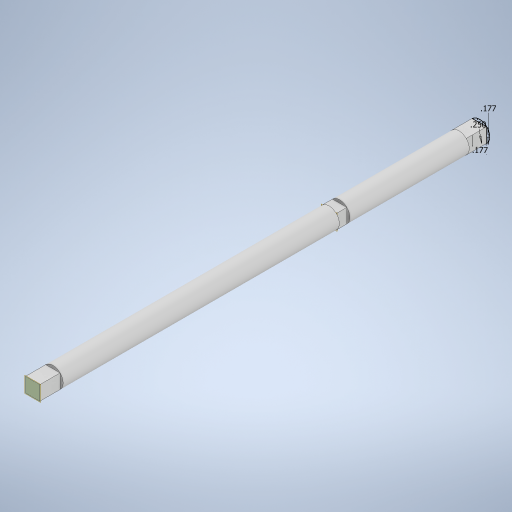
# Autodesk Inventor part: rod
Saved by Autodesk Inventor 2023 (Build 270158000, 158)
## iProperties
Created: 2023-11-14
Part Number: rod
Material: Generic
Document SubType Name: Modeling
Designer: Nate
Density: 1 g/cm^3
Appearance: Default
Author: Nate
Autodesk Inventor part; units mm, degrees
ref_plane "YZ Plane" through (0, 0, 0) normal (1, 0, 0) x (0, 1, 0)
ref_plane "XZ Plane" through (0, 0, 0) normal (0, 1, 0) x (-1, 0, 0)
ref_plane "XY Plane" through (0, 0, 0) normal (0, 0, 1) x (1, 0, 0)
sketch "Sketch1" plane through (0, 0, 0) normal (0, 0, 1) x (1, 0, 0)
  circle A0 centre (0, 0) radius 3.175
  line L0 (-2.2451, 2.2451) -> (2.2451, 2.2451)
  line L1 (2.2451, 2.2451) -> (2.2451, -2.2451)
  line L2 (2.2451, -2.2451) -> (-2.2451, -2.2451)
  line L3 (-2.2451, -2.2451) -> (-2.2451, 2.2451)
  line L4 (-2.2451, 2.2451) -> (2.2451, -2.2451) construction
  line L5 (2.2451, 2.2451) -> (-2.2451, -2.2451) construction
  dimension "d0" = 6.35
  dimension "d6" = 4.4901
  dimension "d7" = 4.4901
  constraints: 12 end point, 2 midpoint, 2 parallel, 1 centre point, 1 coincident, 1 horizontal, 1 perpendicular
  measures "d0" diameter of A0
  measures "d6" distance between parallel lines of L1 L3
  measures "d7" distance between parallel lines of L0 L2
extrude "Extrusion1" add sketch "Sketch1" along normal blind 139.7
extrude "Extrusion2" cut sketch "Sketch1" along normal blind 6.35 contours A0 L1 | L0 A0 | A0 L2 | L3 A0
ref_plane "Work Plane1" through (0, 0, 139.7) normal (0, 0, -1) x (-1, 0, 0)
sketch "Sketch2" plane through (0, 0, 139.7) normal (0, 0, -1) x (-1, 0, 0)
  line L0 (-2.2451, 2.2451) -> (-2.2451, -2.2451) projected
  line L1 (2.2451, 2.2451) -> (-2.2451, 2.2451)
  line L2 (-2.2451, 2.2451) -> (-2.2451, -2.2451)
  line L3 (-2.2451, -2.2451) -> (2.2451, -2.2451)
  line L4 (2.2451, -2.2451) -> (2.2451, 2.2451)
  line L5 (2.2451, 2.2451) -> (-2.2451, -2.2451) construction
  line L6 (-2.2451, 2.2451) -> (2.2451, -2.2451) construction
  circle A0 centre (0, 0) radius 3.175
  dimension "d11" = 4.4901
  dimension "d12" = 4.4901
  dimension "d13" = 6.35
  constraints: 12 end point, 2 midpoint, 2 parallel, 1 centre point, 1 coincident, 1 horizontal, 1 perpendicular
  measures "d11" distance of L3.end L0.end
  measures "d12" distance of L0.end L1.end
  measures "d13" diameter of A0
extrude "Extrusion3" cut sketch "Sketch2" along normal blind 6.35 contours A0 L1 | L0 A0 | L3 A0 | A0 L4
ref_plane "Work Plane2" through (0, 0, 46.99) normal (0, 0, 1) x (1, 0, 0)
sketch "Sketch3" plane through (0, 0, 46.99) normal (0, 0, 1) x (1, 0, 0)
  circle A0 centre (0, 0) radius 3.175
  line L0 (-2.2451, 2.2451) -> (2.2451, 2.2451)
  line L1 (2.2451, 2.2451) -> (2.2451, -2.2451)
  line L2 (2.2451, -2.2451) -> (-2.2451, -2.2451)
  line L3 (-2.2451, -2.2451) -> (-2.2451, 2.2451)
  line L4 (-2.2451, 2.2451) -> (2.2451, -2.2451) construction
  line L5 (2.2451, 2.2451) -> (-2.2451, -2.2451) construction
  dimension "d17" = 4.4901
  dimension "d18" = 4.4901
  constraints: 12 end point, 2 midpoint, 2 parallel, 1 centre point, 1 coincident, 1 horizontal, 1 perpendicular
  measures "d17" distance of L1.end L2.end
  measures "d18" distance of L0.end L1.end
extrude "Extrusion4" cut sketch "Sketch3" against normal blind 3.302 contours A0 L1 | L0 A0 | A0 L2 | L3 A0
body "Solid1"
